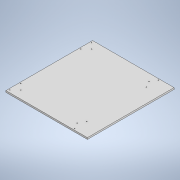
# Autodesk Inventor part: MDFBase
Saved by Autodesk Inventor 2022 (Build 260153000, 153)
## iProperties
Created: 2021-06-29
Part Number: MDFBase
Material: Generic
Document SubType Name: Modeling
Designer: BBL
Density: 1 g/cm^3
Appearance: Default
Author: BBL
Autodesk Inventor part; units mm, degrees
ref_plane "YZ Plane" through (0, 0, 0) normal (1, 0, 0) x (0, 1, 0)
ref_plane "XZ Plane" through (0, 0, 0) normal (0, 1, 0) x (-1, 0, 0)
ref_plane "XY Plane" through (0, 0, 0) normal (0, 0, 1) x (1, 0, 0)
sketch "Sketch1" plane through (0, 0, 0) normal (0, 1, 0) x (-1, 0, 0)
  line L0 (0, 0) -> (600, 0)
  line L1 (600, 0) -> (600, -638)
  line L2 (600, -638) -> (0, -638)
  line L3 (0, -638) -> (0, 0)
  circle A0 centre (104.75, -628) radius 2.75
  circle A1 centre (104.75, -539) radius 2.75
  circle A2 centre (129.75, -583.5) radius 2.75
  circle A3 centre (590, -620) radius 2.75
  circle A4 centre (590, -540) radius 2.75
  circle A5 centre (548.9, -580) radius 2.75
  line L4 (0, -319) -> (600, -319) construction
  circle A6 centre (104.75, -10) radius 2.75
  circle A7 centre (104.75, -99) radius 2.75
  circle A8 centre (129.75, -54.5) radius 2.75
  circle A9 centre (590, -18) radius 2.75
  circle A10 centre (590, -98) radius 2.75
  circle A11 centre (548.9, -58) radius 2.75
  dimension "d0" = 638
  dimension "d1" = 600
  dimension "d4" = 5.5
  dimension "d5" = 495.25
  dimension "d6" = 10
  dimension "d7" = 5.5
  dimension "d8" = 89
  dimension "d9" = 495.25
  dimension "d10" = 5.5
  dimension "d11" = 44.5
  dimension "d12" = 25
  dimension "d13" = 5.5
  dimension "d14" = 10
  dimension "d15" = 18
  dimension "d16" = 5.5
  dimension "d17" = 5.5
  dimension "d18" = 80
  dimension "d19" = 10
  dimension "d20" = 40
  dimension "d21" = 41.1
  constraints: 12 centre point, 10 end point, 6 symmetric about line, 2 midpoint, 2 parallel, 1 horizontal, 1 perpendicular, 6 other
  measures "d0" distance of L0.end L1.end
  measures "d1" distance of L1.end L2.end
  measures "d4" diameter of A0
  measures "d5" distance from line of L1 A0.centre
  measures "d6" distance from line of L2 A0.centre
  measures "d7" diameter of A1
  measures "d8" distance of A0.centre A1.centre
  measures "d9" distance from line of L1 A1.centre
  measures "d10" diameter of A2
  measures "d11" vertical distance of A0.centre A2.centre
  measures "d12" horizontal distance of A0.centre A2.centre
  measures "d13" diameter of A3
  measures "d14" distance from line of L1 A3.centre
  measures "d15" distance from line of L2 A3.centre
  measures "d16" diameter of A4
  measures "d17" diameter of A5
  measures "d18" distance of A3.centre A4.centre
  measures "d19" distance from line of L1 A4.centre
  measures "d20" vertical distance of A4.centre A5.centre
  measures "d21" horizontal distance of A4.centre A5.centre
extrude "Extrusion1" add sketch "Sketch1" along normal blind 12
equation "\"d9\" = d5"
equation "\"d11\" = 0.5 * d8"
equation "\"d19\" = d14"
equation "\"d20\" = 0.5 * d18"
body "Solid1"
